Autodesk Fusion 360 part; units mm, degrees
(part 2 of 2)
sketch "Sketch3" plane through (0, 0, 1.6) normal (0, 0, 1) x (-1, 0, 0)
  line L0 (2.2, 0.2901) -> (2.2, -2.4)
  line L1 (2.2, -2.4) -> (-0.9, -2.4)
  line L2 (-0.9, -2.4) -> (-0.9, 0.2901)
  line L3 (-0.9, 0.2901) -> (2.2, 0.2901)
  circle A0 centre (-2.5972, -6.3613) radius 0.375
  circle A1 centre (-5.1272, 4.1387) radius 0.375
  circle A2 centre (-7.7272, -6.3613) radius 0.375
  circle A3 centre (5.1728, 4.1387) radius 0.375
  circle A4 centre (2.5228, 4.1387) radius 0.375
  circle A5 centre (-5.1672, -6.3613) radius 0.375
  circle A6 centre (-0.0272, 4.1387) radius 0.375
  circle A7 centre (-2.5772, 4.1387) radius 0.375
  circle A8 centre (-0.0372, -6.3613) radius 0.375
  circle A9 centre (2.5328, -6.3613) radius 0.375
  circle A10 centre (7.6728, -6.3613) radius 0.375
  circle A11 centre (6.9478, 1.3137) radius 1.5
  circle A12 centre (5.1028, -6.3613) radius 0.375
  circle A13 centre (-7.0022, 1.3137) radius 1.5
  arc A14 (7.9478, -7.7363) -> (8.9478, -6.7363) centre (7.9478, -6.7363) ccw
  line L4 (8.9478, -6.7363) -> (8.9478, 4.5137)
  arc A15 (8.9478, 4.5137) -> (7.9478, 5.5137) centre (7.9478, 4.5137) ccw
  line L5 (7.9478, 5.5137) -> (-8.0022, 5.5137)
  arc A16 (-8.0022, 5.5137) -> (-9.0022, 4.5137) centre (-8.0022, 4.5137) ccw
  line L6 (-9.0022, 4.5137) -> (-9.0022, -6.7363)
  arc A17 (-9.0022, -6.7363) -> (-8.0022, -7.7363) centre (-8.0022, -6.7363) ccw
  line L7 (-8.0022, -7.7363) -> (7.9478, -7.7363)
  circle A18 centre (-7.7272, -6.3613) radius 0.875
  circle A19 centre (-5.1672, -6.3613) radius 0.875
  circle A20 centre (-2.5972, -6.3613) radius 0.875
  circle A21 centre (-0.0372, -6.3613) radius 0.875
  circle A22 centre (2.5328, -6.3613) radius 0.875
  circle A23 centre (5.1028, -6.3613) radius 0.875
  circle A24 centre (7.6728, -6.3613) radius 0.875
  circle A25 centre (5.1728, 4.1387) radius 0.875
  circle A26 centre (2.5228, 4.1387) radius 0.875
  circle A27 centre (-0.0272, 4.1387) radius 0.875
  circle A28 centre (-2.5772, 4.1387) radius 0.875
  circle A29 centre (-5.1272, 4.1387) radius 0.875
extrude "Extrude3" cut sketch "Sketch3" against normal blind 0.01 contours A18 | A19 | A20 | A21 | A22 | A23 | A24 | A25 | A26 | A27 | A28 | A29
